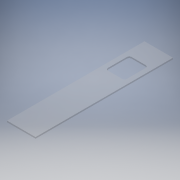
# Autodesk Inventor part: Schläuse
Saved by Autodesk Inventor 2018 (Build 220112000, 112)
## iProperties
Created: 2013-02-21
Part Number: Schläuse
Material: Polycarbonate, Clear
Document SubType Name: Modeling
Designer: Neef
Mass: 592.561 g
Surface Area: 1495.34 cm^2
Volume: 423.258 cm^3
Density: 1.2 g/cm^3
Appearance: Polycarbonate - Clear
Author: Neef
Autodesk Inventor part; units mm, degrees
ref_plane "YZ Plane" through (0, 0, 0) normal (1, 0, 0) x (0, 1, 0)
ref_plane "XZ Plane" through (0, 0, 0) normal (0, 1, 0) x (-1, 0, 0)
ref_plane "XY Plane" through (0, 0, 0) normal (0, 0, 1) x (1, 0, 0)
sketch "Skizze1" plane through (0, 0, 0) normal (0, 0, 1) x (1, 0, 0)
  line L0 (0, 408.1) -> (0, -408.1) projected
  line L1 (-84.7, 0) -> (84.7, 0) projected
  line L2 (-60.5, -291.5) -> (60.5, -291.5)
  line L3 (60.5, -291.5) -> (60.5, 291.5)
  line L4 (60.5, 291.5) -> (-60.5, 291.5)
  line L5 (-60.5, 291.5) -> (-60.5, -291.5)
  point P0 (0, 0)
  point P1 (0, -291.5)
  point P2 (-60.5, 0)
  dimension "d0" = 583
  dimension "d1" = 121
  constraints: 8 end point, 2 midpoint, 2 parallel, 2 point on line, 1 horizontal, 1 perpendicular
  measures "d0" distance of L4.end L2.start
  measures "d1" distance of L2.start L2.end
extrude "Extrusion1" add sketch "Skizze1" along normal blind 6
sketch "Skizze2" plane through (0, 0, 0) normal (0, 0, -1) x (-1, 0, 0)
  line L0 (60.5, 291.5) -> (60.5, -291.5) projected
  line L1 (-60.5, 291.5) -> (60.5, 291.5) projected
  line L2 (-40, 106.5) -> (40, 106.5)
  line L3 (40, 106.5) -> (40, 206.5)
  line L4 (40, 206.5) -> (-40, 206.5)
  line L5 (-40, 206.5) -> (-40, 106.5)
  line L6 (50, 227.269) -> (50, 127.269) projected
  point P0 (0, 0)
  dimension "d4" = 185
  dimension "d5" = 100
  dimension "d6" = 80
  dimension "d7" = 20.5
  constraints: 8 end point, 2 parallel, 1 horizontal, 1 perpendicular
  measures "d4" distance between parallel lines of L1 L2
  measures "d5" distance of L2.end L3.end
  measures "d6" distance of L3.end L4.end
  measures "d7" distance between parallel lines of L0 L3
extrude "Extrusion2" cut sketch "Skizze2" against normal through all
fillet "Rundung1" radius 10 4 edges at (-40, 106.5, 3) (-40, 206.5, 3) (40, 206.5, 3) (40, 106.5, 3)
